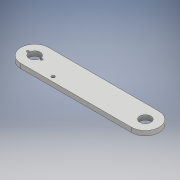
# Autodesk Inventor part: idlerMount
Saved by Autodesk Inventor 2018.3 (Build 223284000, 284)
## iProperties
Created: 2018-06-21
Part Number: idlerMount
Material: Generic
Document SubType Name: Modeling
Designer: mzhang
Density: 1 g/cm^3
Appearance: Default
Author: mzhang
Autodesk Inventor part; units mm, degrees
ref_plane "YZ Plane" through (0, 0, 0) normal (1, 0, 0) x (0, 1, 0)
ref_plane "XZ Plane" through (0, 0, 0) normal (0, 1, 0) x (-1, 0, 0)
ref_plane "XY Plane" through (0, 0, 0) normal (0, 0, 1) x (1, 0, 0)
sketch "Sketch1" plane through (0, 0, 0) normal (0, 0, 1) x (1, 0, 0)
  circle A0 centre (0, 0) radius 6
  arc A1 (0, 15) -> (0, -15) centre (0, 0) ccw
  line L0 (0, 15) -> (120, 15)
  line L1 (0, -15) -> (120, -15)
  arc A2 (120, -15) -> (120, 15) centre (120, 0) ccw
  circle A3 centre (120, 0) radius 6
  dimension "d0" = 12
  dimension "d1" = 30
  dimension "d2" = 120
  dimension "d6" = 120
  dimension "d9" = 12
  constraints: 4 centre point, 4 end point, 4 point on circle, 3 coincident, 2 horizontal, 2 tangent
  measures "d0" diameter of A0
  measures "d1" diameter of A1
  measures "d2" distance of L0.start L0.end
  measures "d6" distance of L1.start L1.end
  measures "d9" diameter of A3
extrude "Extrusion1" add sketch "Sketch1" along normal blind 5
sketch "Sketch2" plane through (0, 0, 5) normal (0, 0, 1) x (1, 0, 0)
  circle A0 centre (30, -10) radius 1.75
  line L0 (0, -15) -> (120, -15) projected
  point P0 (0, 0)
  dimension "d10" = 3.5
  dimension "d11" = 5
  dimension "d15" = 30
  constraints: 1 centre point
  measures "d10" diameter of A0
  measures "d11" distance from line of L0 A0.centre
  measures "d15" horizontal distance of L0.start A0.centre
extrude "Extrusion2" cut sketch "Sketch2" against normal up to surface (5 mm away)
sketch "Sketch3" plane through (0, 0, 5) normal (0, 0, 1) x (1, 0, 0)
  circle A0 centre (0, 0) radius 6 projected
  circle A1 centre (0, 0) radius 7.4422
  circle A2 centre (7.4422, 0) radius 1.25
  circle A3 centre (-7.4422, 0) radius 1.25
  dimension "d16" = 14.8844
  dimension "d17" = 2.5
  dimension "d18" = 2.5
  constraints: 3 centre point, 2 point on circle, 1 coincident
  measures "d16" diameter of A1
  measures "d17" diameter of A2
  measures "d18" diameter of A3
extrude "Extrusion3" cut sketch "Sketch3" against normal up to surface (5 mm away) contours A1 A2 | A1 A2 | A3 A1 | A1 A3
body "Solid1"
